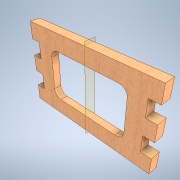
# Autodesk Inventor part: Front
Saved by Autodesk Inventor 2021.2 (Build 252289000, 289)
## iProperties
Created: 2021-03-04
Part Number: Front
Material: Wood (Cherry)
Document SubType Name: Modeling
Designer: 443201246
Density: 0.63 g/cm^3
Appearance: Cherry - Natural Low Gloss
Author: 443201246
Autodesk Inventor part; units mm, degrees
ref_plane "YZ Plane" through (0, 0, 0) normal (1, 0, 0) x (0, 1, 0)
ref_plane "XZ Plane" through (0, 0, 0) normal (0, 1, 0) x (-1, 0, 0)
ref_plane "XY Plane" through (0, 0, 0) normal (0, 0, 1) x (1, 0, 0)
sketch "Sketch1" plane through (0, 0, 0) normal (0, 0, 1) x (1, 0, 0)
  line L0 (0, 0) -> (164, 0)
  line L1 (164, 0) -> (164, 100)
  line L2 (164, 100) -> (0, 100)
  line L3 (0, 100) -> (0, 0)
  dimension "d0" = 164
  dimension "d1" = 100
  constraints: 8 end point, 2 parallel, 1 horizontal, 1 perpendicular
  measures "d0" distance of L2.end L1.end
  measures "d1" distance of L1.end L0.end
extrude "Extrusion1" add sketch "Sketch1" along normal blind 12
sketch "Sketch2" plane through (0, 0, 12) normal (0, 0, 1) x (1, 0, 0)
  line L0 (0, 100) -> (0, 0) projected
  line L1 (164, 100) -> (0, 100) projected
  line L2 (0, 100) -> (0, 0) projected
  line L3 (0, 20) -> (12, 20)
  line L4 (12, 20) -> (12, 40)
  line L5 (12, 40) -> (0, 40)
  line L6 (0, 40) -> (0, 20)
  line L7 (0, 0) -> (164, 0) projected
  line L8 (0, 60) -> (12, 60)
  line L9 (12, 60) -> (12, 80)
  line L10 (12, 80) -> (0, 80)
  line L11 (0, 80) -> (0, 60)
  point P0 (0, 40)
  dimension "d7" = 12
  dimension "d8" = 20
  dimension "d9" = 20
  dimension "d10" = 12
  dimension "d11" = 20
  dimension "d12" = 20
  constraints: 16 end point, 4 parallel, 2 horizontal, 2 perpendicular, 2 point on line
  measures "d7" distance of L5.end L4.end
  measures "d8" distance of L4.end L3.end
  measures "d9" distance between parallel lines of L3 L7
  measures "d10" distance of L10.end L9.end
  measures "d11" distance of L9.end L8.end
  measures "d12" distance between parallel lines of L8 L5
extrude "Extrusion2" cut sketch "Sketch2" against normal through all
ref_plane "Work Plane1" through (82, 0, 0) normal (1, 0, 0) x (0, 0, -1)
mirror "Mirror1" about plane through (82, 0, 0) normal (1, 0, 0) of "Extrusion2"
sketch "Sketch3" plane through (0, 0, 12) normal (0, 0, 1) x (1, 0, 0)
  line L0 (42, 20) -> (122, 20)
  line L1 (132, 30) -> (132, 70)
  line L2 (122, 80) -> (42, 80)
  line L3 (32, 70) -> (32, 30)
  line L4 (0, 0) -> (164, 0) projected
  line L5 (0, 60) -> (0, 40) projected
  arc A0 (42, 80) -> (32, 70) centre (42, 70) ccw
  arc A1 (132, 70) -> (122, 80) centre (122, 70) ccw
  arc A2 (122, 20) -> (132, 30) centre (122, 30) ccw
  arc A3 (32, 30) -> (42, 20) centre (42, 30) ccw
  point P0 (132, 80)
  point P1 (132, 20)
  point P2 (32, 80)
  dimension "d15" = 100
  dimension "d16" = 60
  dimension "d17" = 20
  dimension "d18" = 32
  dimension "d19" = 10
  constraints: 8 end point, 8 point on circle, 8 tangent, 6 point on line, 4 centre point, 3 equal radius, 2 parallel, 1 horizontal, 1 perpendicular
  measures "d15" distance of point (32, 80) point (132, 80)
  measures "d16" distance of point (132, 80) point (132, 20)
  measures "d17" distance between parallel lines of L4 L0
  measures "d18" distance between parallel lines of L5 L3
  measures "d19" radius of A0
extrude "Extrusion3" cut sketch "Sketch3" against normal through all
sketch "Sketch4" plane through (0, 0, 0) normal (0, 0, -1) x (-1, 0, 0)
  line L0 (-122, 80) -> (-42, 80) projected
  arc A0 (-32, 70) -> (-42, 80) centre (-42, 70) ccw projected
  line L1 (-32, 70) -> (-32, 30) projected
  arc A1 (-42, 20) -> (-32, 30) centre (-42, 30) ccw projected
  line L2 (-42, 20) -> (-122, 20) projected
  arc A2 (-132, 30) -> (-122, 20) centre (-122, 30) ccw projected
  line L3 (-132, 30) -> (-132, 70) projected
  arc A3 (-122, 80) -> (-132, 70) centre (-122, 70) ccw projected
  line L4 (-42, 88) -> (-122, 88)
  arc A4 (-122, 88) -> (-140, 70) centre (-122, 70) ccw
  line L5 (-140, 70) -> (-140, 30)
  arc A5 (-140, 30) -> (-122, 12) centre (-122, 30) ccw
  line L6 (-122, 12) -> (-42, 12)
  arc A6 (-42, 12) -> (-24, 30) centre (-42, 30) ccw
  line L7 (-24, 30) -> (-24, 70)
  arc A7 (-24, 70) -> (-42, 88) centre (-42, 70) ccw
  point P0 (0, 0)
  dimension "d22" = 8
  constraints: 8 end point, 8 point on circle, 4 centre point, 7 other
  measures "d22" distance between parallel lines of L0 L4
extrude "Extrusion4" cut sketch "Sketch4" against normal blind 3
body "Solid1"
